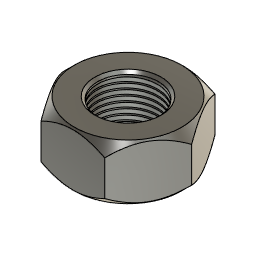
Hex Nut (Autodesk Fusion 360 design; units mm, degrees)
Autodesk Fusion 360 part; units mm, degrees
sketch "Sketch1" plane through (0, 0, 0) normal (0, 0, 1) x (1, 0, 0)
  line L0 (-5.7735, 10) -> (-11.547, 0)
  line L1 (-11.547, 0) -> (-5.7735, -10)
  line L2 (-5.7735, -10) -> (5.7735, -10)
  line L3 (5.7735, -10) -> (11.547, 0)
  line L4 (11.547, 0) -> (5.7735, 10)
  line L5 (5.7735, 10) -> (-5.7735, 10)
  dimension "d1" = 10
  measures "d1" distance of origin L5
extrude "Extrude1" add sketch "Sketch1" along normal blind 10
sketch "Sketch2" plane through (0, 0, 0) normal (0, 1, 0) x (1, 0, 0)
  line L0 (5.7735, -10) -> (11.547, -10)
  line L1 (11.547, -10) -> (9.747, -10)
  line L2 (11.547, -10) -> (11.547, -8.2)
  line L3 (9.747, -10) -> (11.547, -8.2)
  point P0 (11.547, -10)
  dimension "d4" = 1.8
  dimension "d5" = 1.8
  constraint coincident P0 L0.end
  constraint parallel L0 L1
  constraint perpendicular L0 L2
  measures "d4" distance of P0 L1.end
  measures "d5" distance of P0 L2.end
revolve "Revolve1" cut sketch "Sketch2" angle 360 about axis through (0, 0, 1.75) along (0, 0, 1)
ref_plane "WorkPlane1" through (0, 0, 5) normal (0, 0, 1) x (1, 0, 0)
mirror "Mirror1" about plane through (0, 0, 5) normal (0, 0, 1) of "Revolve1"
hole "Hole1" at (0, 0, 10) direction (0, 0, -1) diameter 10.274 depth 10 tip angle 180 countersink diameter 12 countersink angle 90
thread "Thread1" "GB Metric profile 12.0 M12x1 6H" major diameter 12.152 minor diameter 11.035 pitch 1 angle 60 modelled right hand crest width 0.2719 on face at (0.2561, -5.1306, 6.0913) crest through (5.5175, 0, 8.887)
